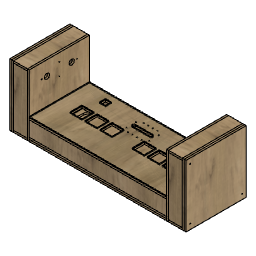
ongekicon-diy (Autodesk Fusion 360 design; units mm, degrees)
Autodesk Fusion 360 part; units mm, degrees
(part 1 of 2)
sketch "스케치1" plane through (0, 0, 0) normal (0, 0, 1) x (1, 0, 0)
  line L0 (289, -642.7336) -> (375, -642.7336)
  line L1 (375, -656.7336) -> (289, -656.7336)
  arc A0 (289, -642.7336) -> (289, -656.7336) centre (289, -649.7336) ccw
  arc A1 (375, -656.7336) -> (375, -642.7336) centre (375, -649.7336) ccw
  line L2 (289, -642.7336) -> (289, -656.7336) construction
  line L3 (375, -642.7336) -> (375, -656.7336) construction
  line L4 (375, -642.7336) -> (386.9217, -626.4866) construction
  line L5 (386.9217, -626.4866) -> (386.9217, -642.6701) construction
  line L6 (386.9217, -642.6701) -> (386.9217, -656.6701) construction
  line L7 (386.9217, -656.6701) -> (386.9217, -672.8535) construction
  line L8 (375, -656.7336) -> (386.9217, -672.8535) construction
  line L9 (386.9217, -642.6701) -> (386.9217, -656.6701) construction
  line L10 (375, -642.7336) -> (375, -656.7336) construction
  line L11 (375, -642.7336) -> (386.9217, -626.4866) construction
  line L12 (375, -656.7336) -> (386.9217, -672.8535) construction
  line L13 (386.9217, -656.6701) -> (386.9217, -672.8535) construction
  line L14 (386.9217, -626.4866) -> (386.9217, -642.6701) construction
  arc A2 (375, -656.7336) -> (375, -642.7336) centre (375, -649.7336) ccw
  line L15 (375, -642.7336) -> (386.9217, -642.7336) construction
  line L16 (289, -642.7336) -> (277.0783, -642.7336) construction
  line L17 (277.0783, -642.7336) -> (277.0783, -626.5501) construction
  line L18 (277.0783, -626.5501) -> (289, -642.7336) construction
  line L19 (289, -656.7336) -> (277.0783, -656.7336) construction
  line L20 (277.0783, -656.7336) -> (277.0783, -672.9171) construction
  line L21 (289, -656.7336) -> (277.0783, -672.9171) construction
  circle A3 centre (277.0783, -626.5501) radius 2.65
  circle A4 centre (277.0783, -672.9171) radius 2.65
  circle A5 centre (386.9217, -626.4866) radius 2.65
  circle A6 centre (386.9217, -672.8535) radius 2.65
  line L22 (299.0783, -611.6097) -> (277.0783, -626.5501) construction
  circle A7 centre (299.0783, -611.6097) radius 2.65
  line L23 (299.0783, -611.6097) -> (321.0783, -611.6097) construction
  line L24 (321.0783, -611.6097) -> (343.0783, -611.6097) construction
  line L25 (343.0783, -611.6097) -> (365.0783, -611.6097) construction
  line L26 (364.9217, -687.7939) -> (386.9217, -672.8535) construction
  line L27 (364.9217, -687.7939) -> (342.9217, -687.7939) construction
  line L28 (342.9217, -687.7939) -> (320.9217, -687.7939) construction
  line L29 (320.9217, -687.7939) -> (298.9217, -687.7939) construction
  circle A8 centre (321.0783, -611.6097) radius 2.65
  circle A9 centre (343.0783, -611.6097) radius 2.65
  circle A10 centre (365.0783, -611.6097) radius 2.65
  circle A11 centre (364.9217, -687.7939) radius 2.65
  circle A12 centre (342.9217, -687.7939) radius 2.65
  circle A13 centre (320.9217, -687.7939) radius 2.65
  circle A14 centre (298.9217, -687.7939) radius 2.65
  line L30 (0, -575) -> (664, -575)
  line L31 (664, -575) -> (664, -866)
  line L32 (664, -866) -> (0, -866)
  line L33 (0, -866) -> (0, -575)
  line L34 (0, -575) -> (332, -575) construction
  line L35 (332, -575) -> (332, -649.7336) construction
  line L36 (0, -649.7336) -> (0, -575) construction
  line L37 (332, -649.7336) -> (289, -649.7336) construction
  line L38 (150.8081, -749.0793) -> (137.915, -749.0793) construction
  line L39 (223.7013, -749.0793) -> (210.8081, -749.0793) construction
  line L40 (0, -1260) -> (664, -1260)
  line L41 (664, -1260) -> (664, -1333)
  line L42 (664, -1333) -> (0, -1333)
  line L43 (0, -1333) -> (0, -1260)
  line L44 (0, -1495) -> (0, -1422)
  line L45 (664, -1422) -> (664, -1495)
  line L46 (0, -1422) -> (664, -1422)
  line L47 (664, -1495) -> (0, -1495)
  line L48 (664, 150) -> (664, -141)
  line L49 (0, -141) -> (0, 150)
  line L50 (664, -141) -> (0, -141)
  line L51 (604, 120) -> (60, 120)
  line L52 (634, -81) -> (634, 90)
  line L53 (30, 90) -> (30, -81)
  line L54 (634, 120) -> (30, -111) construction
  line L55 (60, -111) -> (604, -111)
  line L56 (0, 150) -> (664, 150)
  line L57 (30, 120) -> (634, -111) construction
  line L58 (0, 120) -> (0, 150) construction
  line L59 (664, -141) -> (644.0002, -121.0002) construction
  line L60 (664, 150) -> (644.0002, 130.0002) construction
  line L61 (0, 150) -> (19.9998, 130.0002) construction
  line L62 (0, -141) -> (19.9998, -121.0002) construction
  line L63 (664, -491) -> (644.0002, -471.0002) construction
  line L64 (664, -200) -> (644.0002, -219.9998) construction
  line L65 (634, -431) -> (634, -260)
  line L66 (664, -200) -> (664, -491)
  line L67 (30, -230) -> (634, -461) construction
  line L68 (0, -200) -> (664, -200)
  line L69 (60, -461) -> (604, -461)
  line L70 (664, -491) -> (0, -491)
  line L71 (634, -230) -> (30, -461) construction
  line L72 (30, -260) -> (30, -431)
  line L73 (0, -491) -> (19.9998, -471.0002) construction
  line L74 (604, -230) -> (60, -230)
  line L75 (0, -491) -> (0, -200)
  line L76 (0, -200) -> (19.9998, -219.9998) construction
  line L77 (0, -230) -> (0, -200) construction
  arc A15 (60, 120) -> (30, 90) centre (60, 90) ccw
  arc A16 (634, 90) -> (604, 120) centre (604, 90) ccw
  arc A17 (604, -111) -> (634, -81) centre (604, -81) ccw
  arc A18 (30, -81) -> (60, -111) centre (60, -81) ccw
  arc A19 (60, -230) -> (30, -260) centre (60, -260) ccw
  arc A20 (634, -260) -> (604, -230) centre (604, -260) ccw
  arc A21 (604, -461) -> (634, -431) centre (604, -431) ccw
  arc A22 (30, -431) -> (60, -461) centre (60, -431) ccw
  circle A23 centre (644.0002, -219.9998) radius 3.25
  circle A24 centre (644.0002, -471.0002) radius 3.25
  circle A25 centre (644.0002, -121.0002) radius 9
  circle A26 centre (644.0002, 130.0002) radius 9
  circle A27 centre (19.9998, 130.0002) radius 9
  circle A28 centre (19.9998, -121.0002) radius 9
  circle A29 centre (19.9998, -219.9998) radius 3.25
  circle A30 centre (19.9998, -471.0002) radius 3.25
  line L78 (664, -575) -> (644, -575) construction
  line L79 (644, -575) -> (644, -595) construction
  line L80 (644, -595) -> (664, -595) construction
  line L81 (664, -595) -> (664, -575) construction
  line L82 (664, -866) -> (644, -866) construction
  line L83 (644, -866) -> (644, -846) construction
  line L84 (644, -846) -> (664, -846) construction
  line L85 (664, -846) -> (664, -866) construction
  line L86 (0, -866) -> (20, -866) construction
  line L87 (20, -866) -> (20, -846) construction
  line L88 (20, -846) -> (0, -846) construction
  line L89 (0, -846) -> (0, -866) construction
  line L90 (0, -575) -> (20, -575) construction
  line L91 (20, -575) -> (20, -595) construction
  line L92 (20, -595) -> (0, -595) construction
  line L93 (0, -595) -> (0, -575) construction
  circle A31 centre (20, -595) radius 2.5 construction
  circle A32 centre (644, -595) radius 2.5 construction
  circle A33 centre (20, -846) radius 2.5 construction
  circle A34 centre (644, -846) radius 2.5 construction
  line L94 (1066.4968, -1645.2647) -> (1357.4968, -1645.2647)
  line L95 (1357.4968, -1645.2647) -> (1357.4968, -1712.2647)
  line L96 (1357.4968, -1712.2647) -> (1066.4968, -1712.2647)
  line L97 (1066.4968, -1712.2647) -> (1066.4968, -1645.2647)
  line L98 (716.4968, -1645.2647) -> (1007.4968, -1645.2647)
  line L99 (1007.4968, -1645.2647) -> (1007.4968, -1712.2647)
  line L100 (1007.4968, -1712.2647) -> (716.4968, -1712.2647)
  line L101 (716.4968, -1712.2647) -> (716.4968, -1645.2647)
  line L102 (1066.4968, -845.2647) -> (1357.4968, -845.2647)
  line L103 (1357.4968, -845.2647) -> (1357.4968, -912.2647)
  line L104 (1357.4968, -912.2647) -> (1066.4968, -912.2647)
  line L105 (1066.4968, -912.2647) -> (1066.4968, -845.2647)
  line L106 (716.4968, -845.2647) -> (1007.4968, -845.2647)
  line L107 (1007.4968, -845.2647) -> (1007.4968, -912.2647)
  line L108 (1007.4968, -912.2647) -> (716.4968, -912.2647)
  line L109 (716.4968, -912.2647) -> (716.4968, -845.2647)
  line L110 (1406.0943, -1345.433) -> (1473.0943, -1345.433)
  line L111 (1473.0943, -1345.433) -> (1473.0943, -1627.433)
  line L112 (1473.0943, -1627.433) -> (1406.0943, -1627.433)
  line L113 (1406.0943, -1627.433) -> (1406.0943, -1345.433)
  line L114 (1573.0943, -1627.433) -> (1506.0943, -1627.433)
  line L115 (1506.0943, -1627.433) -> (1506.0943, -1345.433)
  line L116 (1506.0943, -1345.433) -> (1573.0943, -1345.433)
  line L117 (1573.0943, -1345.433) -> (1573.0943, -1627.433)
  line L118 (1506.0943, -1277.433) -> (1506.0943, -995.433)
  line L119 (1506.0943, -995.433) -> (1573.0943, -995.433)
  line L120 (1573.0943, -995.433) -> (1573.0943, -1277.433)
  line L121 (1573.0943, -1277.433) -> (1506.0943, -1277.433)
  line L122 (1406.0943, -1277.433) -> (1406.0943, -995.433)
  line L123 (1406.0943, -995.433) -> (1473.0943, -995.433)
  line L124 (1473.0943, -1277.433) -> (1406.0943, -1277.433)
  line L125 (1473.0943, -995.433) -> (1473.0943, -1277.433)
  line L126 (725.4968, -1278.433) -> (716.4968, -1278.433)
  line L127 (998.4968, -1278.433) -> (725.4968, -1278.433)
  line L128 (998.4968, -1278.433) -> (1007.4968, -1278.433)
  line L129 (1007.4968, -978.433) -> (1007.4968, -1278.433)
  line L130 (1007.4968, -978.433) -> (716.4968, -978.433)
  line L131 (716.4968, -978.433) -> (716.4968, -1278.433)
  arc A35 (1661.5009, -1535.9592) -> (1691.5009, -1565.9592) centre (1691.5009, -1535.9592) ccw
  line L132 (1871.5009, -1325.9592) -> (1691.5009, -1325.9592)
  arc A36 (1691.5009, -1325.9592) -> (1661.5009, -1355.9592) centre (1691.5009, -1355.9592) ccw
  line L133 (1661.5009, -1355.9592) -> (1661.5009, -1535.9592)
  circle A37 centre (1656.0009, -1571.4592) radius 3.25
  circle A38 centre (1656.0009, -1320.4592) radius 3.25
  line L134 (1636.0009, -1295.9592) -> (1636.0009, -1595.9592)
  arc A39 (2251.5009, -1355.9592) -> (2221.5009, -1325.9592) centre (2221.5009, -1355.9592) ccw
  arc A40 (2221.5009, -1565.9592) -> (2251.5009, -1535.9592) centre (2221.5009, -1535.9592) ccw
  circle A41 centre (2257.0009, -1571.4592) radius 10
  circle A42 centre (2257.0009, -1320.4592) radius 10
  circle A43 centre (2006.0009, -1571.4592) radius 10
  line L135 (2221.5009, -1325.9592) -> (2041.5009, -1325.9592)
  circle A44 centre (2006.0009, -1320.4592) radius 10
  line L136 (2041.5009, -1565.9592) -> (2221.5009, -1565.9592)
  line L137 (2277.0009, -1295.9592) -> (2277.0009, -1595.9592)
  arc A45 (2011.5009, -1535.9592) -> (2041.5009, -1565.9592) centre (2041.5009, -1535.9592) ccw
  arc A46 (2041.5009, -1325.9592) -> (2011.5009, -1355.9592) centre (2041.5009, -1355.9592) ccw
  line L138 (2251.5009, -1535.9592) -> (2251.5009, -1355.9592)
  line L139 (2011.5009, -1355.9592) -> (2011.5009, -1535.9592)
  line L140 (1986.0009, -1295.9592) -> (1986.0009, -1595.9592)
  line L141 (1927.0009, -1295.9592) -> (1927.0009, -1595.9592)
  line L142 (1901.5009, -1535.9592) -> (1901.5009, -1355.9592)
  line L143 (1691.5009, -1565.9592) -> (1871.5009, -1565.9592)
  arc A47 (1871.5009, -1565.9592) -> (1901.5009, -1535.9592) centre (1871.5009, -1535.9592) ccw
  arc A48 (1901.5009, -1355.9592) -> (1871.5009, -1325.9592) centre (1871.5009, -1355.9592) ccw
  circle A49 centre (1907.0009, -1320.4592) radius 3.25
  circle A50 centre (1907.0009, -1571.4592) radius 3.25
  line L144 (1927.0009, -1295.9592) -> (1636.0009, -1295.9592)
  line L145 (1927.0009, -1595.9592) -> (1636.0009, -1595.9592)
  line L146 (2277.0009, -1595.9592) -> (1986.0009, -1595.9592)
  line L147 (2277.0009, -1295.9592) -> (1986.0009, -1295.9592)
  line L148 (1927.0009, -1245.9592) -> (1636.0009, -1245.9592)
  line L149 (1927.0009, -945.9592) -> (1927.0009, -1245.9592)
  line L150 (1661.5009, -1005.9592) -> (1661.5009, -1185.9592)
  line L151 (1636.0009, -945.9592) -> (1636.0009, -1245.9592)
  arc A51 (1901.5009, -1005.9592) -> (1871.5009, -975.9592) centre (1871.5009, -1005.9592) ccw
  circle A52 centre (1907.0009, -1221.4592) radius 3.25
  circle A53 centre (1656.0009, -970.4592) radius 3.25
  circle A54 centre (1907.0009, -970.4592) radius 3.25
  line L152 (2277.0009, -945.9592) -> (2277.0009, -1245.9592)
  line L153 (2041.5009, -1215.9592) -> (2221.5009, -1215.9592)
  line L154 (2277.0009, -945.9592) -> (1986.0009, -945.9592)
  line L155 (1691.5009, -1215.9592) -> (1871.5009, -1215.9592)
  line L156 (1901.5009, -1185.9592) -> (1901.5009, -1005.9592)
  arc A55 (1871.5009, -1215.9592) -> (1901.5009, -1185.9592) centre (1871.5009, -1185.9592) ccw
  line L157 (1871.5009, -975.9592) -> (1691.5009, -975.9592)
  line L158 (1986.0009, -945.9592) -> (1986.0009, -1245.9592)
  circle A56 centre (1656.0009, -1221.4592) radius 3.25
  arc A57 (1661.5009, -1185.9592) -> (1691.5009, -1215.9592) centre (1691.5009, -1185.9592) ccw
  arc A58 (1691.5009, -975.9592) -> (1661.5009, -1005.9592) centre (1691.5009, -1005.9592) ccw
  line L159 (1927.0009, -945.9592) -> (1636.0009, -945.9592)
  arc A59 (2011.5009, -1185.9592) -> (2041.5009, -1215.9592) centre (2041.5009, -1185.9592) ccw
  circle A60 centre (2257.0009, -970.4592) radius 10
  circle A61 centre (2006.0009, -1221.4592) radius 10
  line L160 (2011.5009, -1005.9592) -> (2011.5009, -1185.9592)
  arc A62 (2041.5009, -975.9592) -> (2011.5009, -1005.9592) centre (2041.5009, -1005.9592) ccw
  circle A63 centre (2257.0009, -1221.4592) radius 10
  circle A64 centre (2006.0009, -970.4592) radius 10
  line L161 (2277.0009, -1245.9592) -> (1986.0009, -1245.9592)
  line L162 (2251.5009, -1185.9592) -> (2251.5009, -1005.9592)
  arc A65 (2221.5009, -1215.9592) -> (2251.5009, -1185.9592) centre (2221.5009, -1185.9592) ccw
  line L163 (2221.5009, -975.9592) -> (2041.5009, -975.9592)
  arc A66 (2251.5009, -1005.9592) -> (2221.5009, -975.9592) centre (2221.5009, -1005.9592) ccw
  line L164 (716.4968, -1317.433) -> (716.4968, -1617.433)
  circle A67 centre (801.9968, -1386.933) radius 12.5
  line L165 (1007.4968, -1317.433) -> (716.4968, -1317.433)
  line L166 (1007.4968, -1617.433) -> (716.4968, -1617.433)
  circle A68 centre (921.9968, -1386.933) radius 12.5
  line L167 (716.4968, -1521.933) -> (716.4968, -1617.433)
  circle A69 centre (946.9968, -1386.933) radius 2.2361
  circle A70 centre (776.9968, -1386.933) radius 2.2592
  circle A71 centre (861.9968, -1416.933) radius 2.2361
  line L168 (1007.4968, -1317.433) -> (1007.4968, -1617.433)
  line L169 (1007.4968, -1521.933) -> (716.4968, -1521.933) construction
  circle A72 centre (861.9968, -1356.933) radius 2.2361
  line L170 (716.4968, -1278.433) -> (736.4968, -1278.433) construction
  line L171 (736.4968, -1278.433) -> (736.4968, -1253.933) construction
  line L172 (736.4968, -1253.933) -> (716.4968, -1253.933) construction
  line L173 (716.4968, -1253.933) -> (716.4968, -1278.433) construction
  line L174 (1007.4968, -1278.433) -> (987.4968, -1278.433) construction
  line L175 (987.4968, -1278.433) -> (987.4968, -1253.933) construction
  line L176 (987.4968, -1253.933) -> (1007.4968, -1253.933) construction
  line L177 (1007.4968, -1253.933) -> (1007.4968, -1278.433) construction
  line L178 (1007.4968, -978.433) -> (987.4968, -978.433) construction
  line L179 (987.4968, -978.433) -> (987.4968, -1002.933) construction
  line L180 (987.4968, -1002.933) -> (1007.4968, -1002.933) construction
  line L181 (1007.4968, -1002.933) -> (1007.4968, -978.433) construction
  circle A73 centre (736.4968, -1253.933) radius 2.5
  circle A74 centre (987.4968, -1253.933) radius 2.5
  circle A75 centre (987.4968, -1002.933) radius 2.5
  circle A76 centre (1086.4968, -1002.933) radius 2.5
  line L182 (1086.4968, -1278.433) -> (1086.4968, -1253.933) construction
  line L183 (1066.4968, -978.433) -> (1066.4968, -1278.433)
  line L184 (1066.4968, -1002.933) -> (1066.4968, -978.433) construction
  line L185 (1337.4968, -1002.933) -> (1357.4968, -1002.933) construction
  line L186 (1337.4968, -1253.933) -> (1357.4968, -1253.933) construction
  line L187 (1066.4968, -1253.933) -> (1066.4968, -1278.433) construction
  line L188 (1086.4968, -1253.933) -> (1066.4968, -1253.933) construction
  circle A77 centre (1086.4968, -1253.933) radius 2.5
  line L189 (1066.4968, -1278.433) -> (1086.4968, -1278.433) construction
  line L190 (1348.4968, -1278.433) -> (1357.4968, -1278.433)
  line L191 (1086.4968, -1002.933) -> (1066.4968, -1002.933) construction
  line L192 (1066.4968, -978.433) -> (1086.4968, -978.433) construction
  line L193 (1357.4968, -1253.933) -> (1357.4968, -1278.433) construction
  line L194 (1357.4968, -1002.933) -> (1357.4968, -978.433) construction
  line L195 (1337.4968, -978.433) -> (1337.4968, -1002.933) construction
  line L196 (1348.4968, -1278.433) -> (1075.4968, -1278.433)
  line L197 (1086.4968, -978.433) -> (1086.4968, -1002.933) construction
  line L198 (1357.4968, -978.433) -> (1337.4968, -978.433) construction
  line L199 (1357.4968, -978.433) -> (1066.4968, -978.433)
  line L200 (1357.4968, -978.433) -> (1357.4968, -1278.433)
  line L201 (1357.4968, -1278.433) -> (1337.4968, -1278.433) construction
  line L202 (1075.4968, -1278.433) -> (1066.4968, -1278.433)
  circle A78 centre (1337.4968, -1253.933) radius 2.5
  circle A79 centre (1337.4968, -1002.933) radius 2.5
  line L203 (1337.4968, -1278.433) -> (1337.4968, -1253.933) construction
  line L204 (0, -1260) -> (166, -1260) construction
  line L205 (166, -1260) -> (166, -1297.5) construction
  line L206 (166, -1297.5) -> (0, -1297.5) construction
  line L207 (0, -1297.5) -> (0, -1260) construction
  line L208 (664, -1260) -> (498, -1260) construction
  line L209 (498, -1260) -> (498, -1297.5) construction
  line L210 (498, -1297.5) -> (664, -1297.5) construction
  line L211 (664, -1297.5) -> (664, -1260) construction
  circle A80 centre (456.3298, -1576.2079) radius 4
  circle A81 centre (547.3298, -1605.2079) radius 4
  line L212 (592.8298, -1576.2079) -> (592.8298, -1605.2079) construction
  circle A82 centre (592.8298, -1590.7079) radius 4
  circle A83 centre (547.3298, -1576.2079) radius 4
  line L213 (410.8298, -1576.2079) -> (592.8298, -1576.2079) construction
  line L214 (365.3298, -1605.2079) -> (365.3298, -1627.2079) construction
  line L215 (410.8298, -1605.2079) -> (365.3298, -1605.2079) construction
  line L216 (410.8298, -1627.2079) -> (410.8298, -1605.2079) construction
  line L217 (410.8298, -1605.2079) -> (410.8298, -1576.2079) construction
  circle A84 centre (410.8298, -1590.7079) radius 4
  circle A85 centre (501.8298, -1590.7079) radius 4
  line L218 (365.3298, -1627.2079) -> (410.8298, -1627.2079) construction
  circle A86 centre (456.3298, -1605.2079) radius 4
  line L219 (592.8298, -1605.2079) -> (410.8298, -1605.2079) construction
  line L220 (592.8298, -1576.2079) -> (638.3298, -1576.2079) construction
  line L221 (638.3298, -1576.2079) -> (638.3298, -1554.2079) construction
  line L222 (638.3298, -1554.2079) -> (592.8298, -1554.2079) construction
  line L223 (592.8298, -1554.2079) -> (592.8298, -1576.2079) construction
  line L224 (521.8298, -1571.2079) -> (481.2298, -1571.2079)
  line L225 (479.3298, -1573.1079) -> (479.3298, -1578.7079)
  line L226 (481.8298, -1581.2079) -> (521.8298, -1581.2079)
  line L227 (524.3298, -1578.7079) -> (524.3298, -1573.7079)
  arc A87 (524.3298, -1573.7079) -> (521.8298, -1571.2079) centre (521.8298, -1573.7079) ccw
  arc A88 (521.8298, -1581.2079) -> (524.3298, -1578.7079) centre (521.8298, -1578.7079) ccw
  arc A89 (479.3298, -1578.7079) -> (481.8298, -1581.2079) centre (481.8298, -1578.7079) ccw
  arc A90 (481.2298, -1571.2079) -> (479.3298, -1573.1079) centre (481.2298, -1573.1079) ccw
  line L228 (365.3298, -1554.2079) -> (638.3298, -1554.2079)
  line L229 (638.3298, -1554.2079) -> (638.3298, -1627.2079)
  line L230 (638.3298, -1627.2079) -> (365.3298, -1627.2079)
  line L231 (365.3298, -1627.2079) -> (365.3298, -1554.2079)
  arc A91 (884.4968, -1545.933) -> (881.9968, -1543.433) centre (881.9968, -1545.933) ccw
  line L232 (884.4968, -1550.933) -> (884.4968, -1545.933)
  line L233 (770.9968, -1577.433) -> (770.9968, -1548.433) construction
  line L234 (881.9968, -1543.433) -> (841.3968, -1543.433)
  arc A92 (881.9968, -1553.433) -> (884.4968, -1550.933) centre (881.9968, -1550.933) ccw
  arc A93 (839.4968, -1550.933) -> (841.9968, -1553.433) centre (841.9968, -1550.933) ccw
  circle A94 centre (816.4968, -1577.433) radius 4
  circle A95 centre (861.9968, -1562.933) radius 4
  line L235 (841.9968, -1553.433) -> (881.9968, -1553.433)
  arc A96 (841.3968, -1543.433) -> (839.4968, -1545.333) centre (841.3968, -1545.333) ccw
  circle A97 centre (816.4968, -1548.433) radius 4
  line L236 (952.9968, -1577.433) -> (770.9968, -1577.433) construction
  line L237 (839.4968, -1545.333) -> (839.4968, -1550.933)
  line L238 (770.9968, -1548.433) -> (952.9968, -1548.433) construction
  circle A98 centre (770.9968, -1562.933) radius 4
  circle A99 centre (952.9968, -1562.933) radius 4
  circle A100 centre (907.4968, -1577.433) radius 4
  circle A101 centre (907.4968, -1548.433) radius 4
  line L239 (952.9968, -1548.433) -> (952.9968, -1577.433) construction
  line L240 (952.9968, -1548.433) -> (1007.4968, -1548.433) construction
  line L241 (1007.4968, -1548.433) -> (1007.4968, -1521.933) construction
  line L242 (1007.4968, -1521.933) -> (952.9968, -1521.933) construction
  line L243 (952.9968, -1521.933) -> (952.9968, -1548.433) construction
  line L244 (770.9968, -1577.433) -> (716.4968, -1577.433) construction
  line L245 (716.4968, -1577.433) -> (716.4968, -1594.933) construction
  line L246 (716.4968, -1594.933) -> (770.9968, -1594.933) construction
  line L247 (770.9968, -1594.933) -> (770.9968, -1577.433) construction
  circle A102 centre (1302.9968, -1562.933) radius 4
  circle A103 centre (1257.4968, -1548.433) radius 4
  line L248 (1357.4968, -1521.933) -> (1302.9968, -1521.933) construction
  arc A104 (1231.9968, -1553.433) -> (1234.4968, -1550.933) centre (1231.9968, -1550.933) ccw
  arc A105 (1234.4968, -1545.933) -> (1231.9968, -1543.433) centre (1231.9968, -1545.933) ccw
  line L249 (1120.9968, -1577.433) -> (1120.9968, -1548.433) construction
  line L250 (1231.9968, -1543.433) -> (1191.3968, -1543.433)
  line L251 (1120.9968, -1603.933) -> (1120.9968, -1577.433) construction
  circle A106 centre (1211.9968, -1562.933) radius 4
  line L252 (1302.9968, -1521.933) -> (1302.9968, -1548.433) construction
  line L253 (1302.9968, -1548.433) -> (1302.9968, -1577.433) construction
  circle A107 centre (1257.4968, -1577.433) radius 4
  line L254 (1357.4968, -1317.433) -> (1357.4968, -1617.433)
  line L255 (1302.9968, -1548.433) -> (1357.4968, -1548.433) construction
  line L256 (1357.4968, -1548.433) -> (1357.4968, -1521.933) construction
  arc A108 (1189.4968, -1550.933) -> (1191.9968, -1553.433) centre (1191.9968, -1550.933) ccw
  circle A109 centre (1120.9968, -1562.933) radius 4
  line L257 (1234.4968, -1550.933) -> (1234.4968, -1545.933)
  circle A110 centre (1211.9968, -1356.933) radius 2.2361
  circle A111 centre (1166.4968, -1548.433) radius 4
  arc A112 (1191.3968, -1543.433) -> (1189.4968, -1545.333) centre (1191.3968, -1545.333) ccw
  line L258 (1189.4968, -1545.333) -> (1189.4968, -1550.933)
  circle A113 centre (1166.4968, -1577.433) radius 4
  circle A114 centre (1211.9968, -1416.933) radius 2.2361
  circle A115 centre (1126.9968, -1386.933) radius 2.2592
  line L259 (1191.9968, -1553.433) -> (1231.9968, -1553.433)
  circle A116 centre (1151.9968, -1386.933) radius 12.5
  line L260 (1357.4968, -1617.433) -> (1066.4968, -1617.433)
  line L261 (1120.9968, -1577.433) -> (1066.4968, -1577.433) construction
  line L262 (1066.4968, -1603.933) -> (1120.9968, -1603.933) construction
  line L263 (1066.4968, -1521.933) -> (1066.4968, -1617.433)
  line L264 (1066.4968, -1577.433) -> (1066.4968, -1603.933) construction
  line L265 (1066.4968, -1317.433) -> (1066.4968, -1617.433)
  line L266 (1302.9968, -1577.433) -> (1120.9968, -1577.433) construction
  line L267 (1357.4968, -1317.433) -> (1066.4968, -1317.433)
  line L268 (1120.9968, -1548.433) -> (1302.9968, -1548.433) construction
  line L269 (1357.4968, -1521.933) -> (1066.4968, -1521.933) construction
  circle A117 centre (1296.9968, -1386.933) radius 2.2361
  circle A118 centre (1271.9968, -1386.933) radius 12.5
  line L270 (278.3298, -1554.2079) -> (232.8298, -1554.2079) construction
  line L271 (121.8298, -1581.2079) -> (161.8298, -1581.2079)
  line L272 (161.8298, -1571.2079) -> (121.2298, -1571.2079)
  line L273 (50.8298, -1576.2079) -> (232.8298, -1576.2079) construction
  line L274 (119.3298, -1573.1079) -> (119.3298, -1578.7079)
  line L275 (278.3298, -1554.2079) -> (278.3298, -1627.2079)
  line L276 (232.8298, -1576.2079) -> (232.8298, -1605.2079) construction
  line L277 (278.3298, -1576.2079) -> (278.3298, -1554.2079) construction
  arc A119 (161.8298, -1581.2079) -> (164.3298, -1578.7079) centre (161.8298, -1578.7079) ccw
  arc A120 (119.3298, -1578.7079) -> (121.8298, -1581.2079) centre (121.8298, -1578.7079) ccw
  line L278 (232.8298, -1554.2079) -> (232.8298, -1576.2079) construction
  line L279 (232.8298, -1576.2079) -> (278.3298, -1576.2079) construction
  circle A121 centre (187.3298, -1576.2079) radius 4
  arc A122 (121.2298, -1571.2079) -> (119.3298, -1573.1079) centre (121.2298, -1573.1079) ccw
  line L280 (164.3298, -1578.7079) -> (164.3298, -1573.7079)
  circle A123 centre (187.3298, -1605.2079) radius 4
  circle A124 centre (141.8298, -1590.7079) radius 4
  arc A125 (164.3298, -1573.7079) -> (161.8298, -1571.2079) centre (161.8298, -1573.7079) ccw
  line L281 (278.3298, -1627.2079) -> (5.3298, -1627.2079)
  circle A126 centre (96.3298, -1576.2079) radius 4
  line L282 (232.8298, -1605.2079) -> (50.8298, -1605.2079) construction
  circle A127 centre (232.8298, -1590.7079) radius 4
  line L283 (50.8298, -1605.2079) -> (5.3298, -1605.2079) construction
  line L284 (5.3298, -1627.2079) -> (5.3298, -1554.2079)
  circle A128 centre (50.8298, -1590.7079) radius 4
  line L285 (50.8298, -1627.2079) -> (50.8298, -1605.2079) construction
  line L286 (5.3298, -1627.2079) -> (50.8298, -1627.2079) construction
  line L287 (50.8298, -1605.2079) -> (50.8298, -1576.2079) construction
  circle A129 centre (96.3298, -1605.2079) radius 4
  line L288 (5.3298, -1554.2079) -> (278.3298, -1554.2079)
  line L289 (5.3298, -1605.2079) -> (5.3298, -1627.2079) construction
  line L290 (138.1898, -635.6975) -> (109.1898, -635.6975)
  line L291 (109.1898, -635.6975) -> (109.1898, -606.6975)
  line L292 (109.1898, -606.6975) -> (138.1898, -606.6975)
  line L293 (138.1898, -606.6975) -> (138.1898, -635.6975)
  line L294 (138.1898, -635.6975) -> (109.1898, -606.6975) construction
  line L295 (109.1898, -635.6975) -> (138.1898, -606.6975) construction
  line L296 (525.8102, -635.6975) -> (554.8102, -635.6975)
  line L297 (554.8102, -635.6975) -> (554.8102, -606.6975)
  line L298 (554.8102, -606.6975) -> (525.8102, -606.6975)
  line L299 (525.8102, -606.6975) -> (525.8102, -635.6975)
  line L300 (525.8102, -635.6975) -> (554.8102, -606.6975) construction
  line L301 (554.8102, -635.6975) -> (525.8102, -606.6975) construction
  line L302 (664, -1216) -> (644, -1216) construction
  line L303 (644, -945) -> (664, -945) construction
  circle A130 centre (644, -1196) radius 2.5 construction
  line L304 (644, -1216) -> (644, -1196) construction
  line L305 (554.8102, -985.6975) -> (525.8102, -956.6975) construction
  line L306 (554.8102, -985.6975) -> (554.8102, -956.6975)
  line L307 (664, -925) -> (644, -925) construction
  line L308 (109.1898, -985.6975) -> (109.1898, -956.6975)
  line L309 (0, -925) -> (20, -925) construction
  line L310 (20, -925) -> (20, -945) construction
  line L311 (138.1898, -956.6975) -> (138.1898, -985.6975)
  line L312 (0, -999.7336) -> (0, -925) construction
  line L313 (525.8102, -956.6975) -> (525.8102, -985.6975)
  line L314 (525.8102, -985.6975) -> (554.8102, -956.6975) construction
  line L315 (525.8102, -985.6975) -> (554.8102, -985.6975)
  circle A131 centre (644, -945) radius 2.5 construction
  line L316 (664, -945) -> (664, -925) construction
  line L317 (664, -925) -> (664, -1216)
  line L318 (644, -925) -> (644, -945) construction
  circle A132 centre (20, -1196) radius 2.5 construction
  line L319 (0, -1216) -> (0, -925)
  line L320 (0, -945) -> (0, -925) construction
  line L321 (109.1898, -956.6975) -> (138.1898, -956.6975)
  line L322 (0, -925) -> (332, -925) construction
  line L323 (0, -1216) -> (20, -1216) construction
  line L324 (20, -1196) -> (0, -1196) construction
  line L325 (0, -1196) -> (0, -1216) construction
  line L326 (20, -1216) -> (20, -1196) construction
  arc A133 (289, -992.7336) -> (289, -1006.7336) centre (289, -999.7336) ccw
  arc A134 (375, -1006.7336) -> (375, -992.7336) centre (375, -999.7336) ccw
  arc A135 (375, -1006.7336) -> (375, -992.7336) centre (375, -999.7336) ccw
  line L327 (138.1898, -985.6975) -> (109.1898, -985.6975)
  circle A136 centre (20, -945) radius 2.5 construction
  line L328 (20, -945) -> (0, -945) construction
  line L329 (109.1898, -985.6975) -> (138.1898, -956.6975) construction
  line L330 (138.1898, -985.6975) -> (109.1898, -956.6975) construction
  line L331 (375, -1006.7336) -> (289, -1006.7336)
  line L332 (664, -1216) -> (0, -1216)
  line L333 (0, -925) -> (664, -925)
  line L334 (289, -992.7336) -> (375, -992.7336)
  line L335 (644, -1196) -> (664, -1196) construction
  line L336 (664, -1196) -> (664, -1216) construction
  line L337 (554.8102, -956.6975) -> (525.8102, -956.6975)
  line L338 (644, 525) -> (644, 505) construction
  circle A137 centre (644, 254) radius 2.5
  line L339 (664, 525) -> (644, 525) construction
  line L340 (644, 505) -> (664, 505) construction
  line L341 (664, 254) -> (664, 234) construction
  line L342 (664, 505) -> (664, 525) construction
  circle A138 centre (644, 505) radius 2.5
  line L343 (644, 234) -> (644, 254) construction
  line L344 (664, 234) -> (644, 234) construction
  line L345 (644, 254) -> (664, 254) construction
  line L346 (664, 525) -> (664, 234)
  line L347 (0, 525) -> (332, 525) construction
  line L348 (0, 525) -> (664, 525)
  line L349 (664, 234) -> (0, 234)
  line L350 (0, 234) -> (0, 525)
  line L351 (20, 234) -> (20, 254) construction
  line L352 (20, 254) -> (0, 254) construction
  line L353 (0, 254) -> (0, 234) construction
  line L354 (0, 234) -> (20, 234) construction
  circle A139 centre (20, 254) radius 2.5
  circle A140 centre (20, 505) radius 2.5
  line L355 (0, 525) -> (20, 525) construction
  line L356 (20, 505) -> (0, 505) construction
  line L357 (20, 525) -> (20, 505) construction
  line L358 (0, 505) -> (0, 525) construction
  line L359 (180.5, -1312) -> (151.5, -1312)
  line L360 (151.5, -1312) -> (151.5, -1283)
  line L361 (151.5, -1283) -> (180.5, -1283)
  line L362 (180.5, -1283) -> (180.5, -1312)
  line L363 (180.5, -1312) -> (151.5, -1283) construction
  line L364 (151.5, -1312) -> (180.5, -1283) construction
  line L365 (318.75, -1303.75) -> (306.25, -1303.75)
  line L366 (306.25, -1303.75) -> (306.25, -1291.25)
  line L367 (306.25, -1291.25) -> (318.75, -1291.25)
  line L368 (318.75, -1291.25) -> (318.75, -1303.75)
  line L369 (318.75, -1303.75) -> (306.25, -1291.25) construction
  line L370 (306.25, -1303.75) -> (318.75, -1291.25) construction
  line L371 (332, -1333) -> (332, -1260) construction
  line L372 (483.5, -1312) -> (512.5, -1312)
  line L373 (512.5, -1312) -> (512.5, -1283)
  line L374 (483.5, -1283) -> (483.5, -1312)
  line L375 (512.5, -1283) -> (483.5, -1283)
  line L376 (357.75, -1303.75) -> (357.75, -1291.25)
  line L377 (357.75, -1291.25) -> (345.25, -1291.25)
  line L378 (345.25, -1303.75) -> (357.75, -1303.75)
  line L379 (345.25, -1291.25) -> (345.25, -1303.75)
  line L380 (136.915, -748.0793) -> (78.915, -748.0793)
  line L381 (78.915, -748.0793) -> (78.915, -690.0793)
  line L382 (78.915, -690.0793) -> (136.915, -690.0793)
  line L383 (136.915, -690.0793) -> (136.915, -748.0793)
  line L384 (136.915, -748.0793) -> (78.915, -690.0793) construction
  line L385 (78.915, -748.0793) -> (136.915, -690.0793) construction
  line L386 (209.8081, -748.0793) -> (151.8081, -748.0793)
  line L387 (151.8081, -748.0793) -> (151.8081, -690.0793)
  line L388 (151.8081, -690.0793) -> (209.8081, -690.0793)
  line L389 (209.8081, -690.0793) -> (209.8081, -748.0793)
  line L390 (209.8081, -748.0793) -> (151.8081, -690.0793) construction
  line L391 (151.8081, -748.0793) -> (209.8081, -690.0793) construction
  line L392 (282.7013, -748.0793) -> (224.7013, -748.0793)
  line L393 (224.7013, -748.0793) -> (224.7013, -690.0793)
  line L394 (224.7013, -690.0793) -> (282.7013, -690.0793)
  line L395 (282.7013, -690.0793) -> (282.7013, -748.0793)
  line L396 (282.7013, -748.0793) -> (224.7013, -690.0793) construction
  line L397 (224.7013, -748.0793) -> (282.7013, -690.0793) construction
  line L398 (512.1919, -690.0793) -> (454.1919, -690.0793)
  line L399 (454.1919, -748.0793) -> (512.1919, -690.0793) construction
  line L400 (527.085, -748.0793) -> (585.085, -748.0793)
  line L401 (512.1919, -748.0793) -> (454.1919, -690.0793) construction
  line L402 (513.1919, -749.0793) -> (526.085, -749.0793) construction
  line L403 (454.1919, -748.0793) -> (512.1919, -748.0793)
  line L404 (585.085, -748.0793) -> (585.085, -690.0793)
  line L405 (381.2987, -690.0793) -> (381.2987, -748.0793)
  line L406 (381.2987, -748.0793) -> (439.2987, -748.0793)
  line L407 (454.1919, -690.0793) -> (454.1919, -748.0793)
  line L408 (527.085, -748.0793) -> (585.085, -690.0793) construction
  line L409 (585.085, -690.0793) -> (527.085, -690.0793)
  line L410 (439.2987, -690.0793) -> (381.2987, -690.0793)
  line L411 (381.2987, -748.0793) -> (439.2987, -690.0793) construction
  line L412 (440.2987, -749.0793) -> (453.1919, -749.0793) construction
  line L413 (585.085, -748.0793) -> (527.085, -690.0793) construction
  line L414 (527.085, -690.0793) -> (527.085, -748.0793)
  line L415 (512.1919, -748.0793) -> (512.1919, -690.0793)
  line L416 (439.2987, -748.0793) -> (381.2987, -690.0793) construction
  line L417 (439.2987, -748.0793) -> (439.2987, -690.0793)
  line L418 (225.4513, -1098.8293) -> (283.4513, -1040.8293) construction
  line L419 (152.5581, -1098.8293) -> (152.5581, -1040.8293)
  line L420 (79.665, -1098.8293) -> (79.665, -1040.8293)
  line L421 (79.665, -1040.8293) -> (137.665, -1040.8293)
  line L422 (137.665, -1098.8293) -> (79.665, -1040.8293) construction
  line L423 (152.5581, -1040.8293) -> (210.5581, -1040.8293)
  line L424 (151.5581, -1099.8293) -> (138.665, -1099.8293) construction
  line L425 (137.665, -1040.8293) -> (137.665, -1098.8293)
  line L426 (79.665, -1098.8293) -> (137.665, -1040.8293) construction
  line L427 (152.5581, -1098.8293) -> (210.5581, -1040.8293) construction
  line L428 (210.5581, -1098.8293) -> (152.5581, -1098.8293)
  line L429 (210.5581, -1098.8293) -> (152.5581, -1040.8293) construction
  line L430 (137.665, -1098.8293) -> (79.665, -1098.8293)
  line L431 (210.5581, -1040.8293) -> (210.5581, -1098.8293)
  line L432 (225.4513, -1098.8293) -> (225.4513, -1040.8293)
  line L433 (283.4513, -1098.8293) -> (225.4513, -1098.8293)
  line L434 (225.4513, -1040.8293) -> (283.4513, -1040.8293)
  line L435 (283.4513, -1040.8293) -> (283.4513, -1098.8293)
  line L436 (283.4513, -1098.8293) -> (225.4513, -1040.8293) construction
  line L437 (224.4513, -1099.8293) -> (211.5581, -1099.8293) construction
  line L438 (332, -925) -> (332, -1216) construction
  line L439 (526.335, -1098.8293) -> (584.335, -1098.8293)
  line L440 (526.335, -1040.8293) -> (526.335, -1098.8293)
  line L441 (526.335, -1098.8293) -> (584.335, -1040.8293) construction
  line L442 (380.5487, -1040.8293) -> (380.5487, -1098.8293)
  line L443 (380.5487, -1098.8293) -> (438.5487, -1098.8293)
  line L444 (439.5487, -1099.8293) -> (452.4419, -1099.8293) construction
  line L445 (453.4419, -1040.8293) -> (453.4419, -1098.8293)
  line L446 (438.5487, -1098.8293) -> (380.5487, -1040.8293) construction
  line L447 (438.5487, -1098.8293) -> (438.5487, -1040.8293)
  line L448 (380.5487, -1098.8293) -> (438.5487, -1040.8293) construction
  line L449 (438.5487, -1040.8293) -> (380.5487, -1040.8293)
  line L450 (511.4419, -1098.8293) -> (511.4419, -1040.8293)
  line L451 (584.335, -1098.8293) -> (526.335, -1040.8293) construction
  line L452 (453.4419, -1098.8293) -> (511.4419, -1098.8293)
  line L453 (584.335, -1098.8293) -> (584.335, -1040.8293)
  line L454 (511.4419, -1098.8293) -> (453.4419, -1040.8293) construction
  line L455 (511.4419, -1040.8293) -> (453.4419, -1040.8293)
  line L456 (512.4419, -1099.8293) -> (525.335, -1099.8293) construction
  line L457 (584.335, -1040.8293) -> (526.335, -1040.8293)
  line L458 (453.4419, -1098.8293) -> (511.4419, -1040.8293) construction
  line L459 (1636.0009, -945.9592) -> (1656.0009, -970.4592)
  line L460 (1656.0009, -970.4592) -> (1656.0009, -945.9592)
  circle A141 centre (736.4968, -1002.933) radius 2.6
  point P0 (332, 4.5)
  point P1 (332, 4.5)
  point P2 (332, -345.5)
  point P3 (332, -345.5)
  point P4 (0, -350)
  point P5 (1781.5009, -1445.9592)
  point P6 (2131.5009, -1445.9592)
  point P7 (2131.5009, -1095.9592)
  point P8 (1781.5009, -1095.9592)
  point P9 (861.9968, -1564.433)
  point P10 (861.9968, -1564.433)
  point P11 (166, -1297.5)
  point P12 (498, -1297.5)
  point P13 (166, -1297.5)
  point P14 (498, -1297.5)
  point P15 (501.8298, -1590.7079)
  point P16 (501.8298, -1576.2079)
  point P17 (861.9968, -1548.433)
  point P18 (861.9968, -1562.933)
  point P19 (1211.9968, -1564.433)
  point P20 (1211.9968, -1548.433)
  point P21 (1211.9968, -1562.933)
  point P22 (1211.9968, -1564.433)
  point P23 (141.8298, -1576.2079)
  point P24 (141.8298, -1590.7079)
  point P25 (540.3102, -621.1975)
  point P26 (253.7013, -719.0793)
  point P27 (107.915, -719.0793)
  point P28 (123.6898, -621.1975)
  point P29 (107.915, -719.0793)
  point P30 (253.7013, -719.0793)
  point P31 (123.6898, -621.1975)
  point P32 (540.3102, -621.1975)
  point P33 (123.6898, -621.1975)
  point P34 (540.3102, -621.1975)
  point P35 (123.6898, -971.1975)
  point P36 (540.3102, -971.1975)
  point P37 (123.6898, -971.1975)
  point P38 (540.3102, -971.1975)
  point P39 (540.3102, -971.1975)
  point P40 (123.6898, -971.1975)
  point P41 (166, -1297.5)
  point P42 (312.5, -1297.5)
  point P43 (312.5, -1297.5)
  point P44 (107.915, -719.0793)
  point P45 (180.8081, -719.0793)
  point P46 (253.7013, -719.0793)
  point P47 (556.085, -719.0793)
  point P48 (410.2987, -719.0793)
  point P49 (556.085, -719.0793)
  point P50 (410.2987, -719.0793)
  point P51 (410.2987, -719.0793)
  point P52 (483.1919, -719.0793)
  point P53 (556.085, -719.0793)
  point P54 (79.665, -1040.8293)
  point P55 (181.5581, -1069.8293)
  point P56 (108.665, -1069.8293)
  point P57 (254.4513, -1069.8293)
  point P58 (254.4513, -1069.8293)
  point P59 (108.665, -1069.8293)
  point P60 (108.665, -1069.8293)
  point P61 (254.4513, -1069.8293)
  point P62 (482.4419, -1069.8293)
  point P63 (555.335, -1069.8293)
  point P64 (555.335, -1069.8293)
  point P65 (409.5487, -1069.8293)
  point P66 (584.335, -1040.8293)
  point P67 (555.335, -1069.8293)
  point P68 (409.5487, -1069.8293)
  point P69 (409.5487, -1069.8293)
  dimension "d11" = 7
  dimension "d12" = 16.1835
  dimension "d13" = 16.1835
  dimension "d14" = 16.1835
  dimension "d15" = 16.1835
  dimension "d16" = 11.9217
  dimension "d17" = 11.9217
  dimension "d19" = 11.9217
  dimension "d22" = 5.3
  dimension "d23" = 5.3
  dimension "d24" = 5.3
  dimension "d25" = 5.3
  dimension "d26" = 5.3
  dimension "d27" = 22
  dimension "d28" = 22
  dimension "d29" = 22
  dimension "d33" = 5.3
  dimension "d34" = 5.3
  dimension "d35" = 5.3
  dimension "d36" = 5.3
  dimension "d37" = 5.3
  dimension "d38" = 5.3
  dimension "d39" = 5.3
  dimension "d43" = 291
  dimension "d63" = 74.7336
  dimension "d64" = 86
  dimension "d65" = 43
  dimension "d83" = 12.8931
  dimension "d84" = 12.8931
  dimension "d85" = 60
  dimension "d194" = 73
  dimension "d195" = 664
  dimension "d196" = 73
  dimension "d350" = 291
  dimension "d352" = 231
  dimension "d357" = 28.284
  dimension "d358" = 28.284
  dimension "d359" = 28.284
  dimension "d360" = 28.284
  dimension "d361" = 664
  dimension "d362" = 291
  dimension "d363" = 231
  dimension "d364" = 28.284
  dimension "d365" = 28.284
  dimension "d366" = 28.284
  dimension "d367" = 28.284
  dimension "d368" = 30
  dimension "d369" = 30
  dimension "d370" = 30
  dimension "d371" = 30
  dimension "d372" = 30
  dimension "d373" = 30
  dimension "d374" = 30
  dimension "d375" = 30
  dimension "d376" = 6.5
  dimension "d377" = 6.5
  dimension "d378" = 18
  dimension "d379" = 18
  dimension "d380" = 18
  dimension "d381" = 18
  dimension "d382" = 6.5
  dimension "d383" = 6.5
  dimension "d384" = 20
  dimension "d385" = 20
  dimension "d387" = 20
  dimension "d389" = 20
  dimension "d390" = 20
  dimension "d391" = 20
  dimension "d392" = 5
  dimension "d393" = 5
  dimension "d394" = 5
  dimension "d395" = 5
  dimension "d537" = 664
  dimension "d553" = 67
  dimension "d554" = 67
  dimension "d555" = 67
  dimension "d556" = 67
  dimension "d807" = 300
  dimension "d858" = 30
  dimension "d859" = 30
  dimension "d860" = 30
  dimension "d861" = 30
  dimension "d862" = 6.5
  dimension "d863" = 6.5
  dimension "d865" = 6.5
  dimension "d876" = 30
  dimension "d877" = 30
  dimension "d878" = 30
  dimension "d879" = 30
  dimension "d880" = 20
  dimension "d881" = 20
  dimension "d882" = 20
  dimension "d883" = 20
  dimension "d884" = 6.5
  dimension "d892" = 30
  dimension "d893" = 30
  dimension "d894" = 30
  dimension "d895" = 30
  dimension "d896" = 6.5
  dimension "d897" = 6.5
  dimension "d898" = 6.5
  dimension "d899" = 30
  dimension "d900" = 30
  dimension "d901" = 30
  dimension "d902" = 30
  dimension "d903" = 20
  dimension "d904" = 20
  dimension "d905" = 20
  dimension "d906" = 20
  dimension "d907" = 6.5
  dimension "d934" = 300
  dimension "d943" = 25
  dimension "d944" = 25
  dimension "d945" = 20
  dimension "d946" = 24.5
  dimension "d947" = 20
  dimension "d948" = 24.5
  dimension "d949" = 20
  dimension "d950" = 24.5
  dimension "d954" = 5
  dimension "d955" = 5
  dimension "d956" = 5
  dimension "d957" = 300
  dimension "d959" = 24.5
  dimension "d961" = 24.5
  dimension "d962" = 20
  dimension "d963" = 24.5
  dimension "d964" = 20
  dimension "d965" = 24.5
  dimension "d966" = 5
  dimension "d967" = 5
  dimension "d968" = 5
  dimension "d969" = 5
  dimension "d981" = 37.5
  dimension "d983" = 37.5
  dimension "d1011" = 8
  dimension "d1012" = 8
  dimension "d1013" = 8
  dimension "d1014" = 8
  dimension "d1015" = 8
  dimension "d1016" = 8
  dimension "d1017" = 8
  dimension "d1018" = 29
  dimension "d1019" = 45.5
  dimension "d1020" = 22
  dimension "d1049" = 182
  dimension "d1050" = 29
  dimension "d1051" = 45.5
  dimension "d1052" = 22
  dimension "d1055" = 2.5
  dimension "d1056" = 1.9
  dimension "d1057" = 273
  dimension "d1058" = 73
  dimension "d1059" = 8
  dimension "d1060" = 8
  dimension "d1061" = 8
  dimension "d1062" = 8
  dimension "d1063" = 8
  dimension "d1064" = 8
  dimension "d1065" = 8
  dimension "d1066" = 29
  dimension "d1069" = 182
  dimension "d1072" = 2.5
  dimension "d1073" = 1.9
  dimension "d1074" = 54.5
  dimension "d1075" = 26.5
  dimension "d1076" = 54.5
  dimension "d1077" = 17.5
  dimension "d1094" = 25
  dimension "d1095" = 25
  dimension "d1096" = 8
  dimension "d1097" = 8
  dimension "d1098" = 8
  dimension "d1099" = 8
  dimension "d1100" = 8
  dimension "d1101" = 8
  dimension "d1102" = 8
  dimension "d1103" = 29
  dimension "d1104" = 182
  dimension "d1105" = 2.5
  dimension "d1106" = 1.9
  dimension "d1107" = 54.5
  dimension "d1108" = 26.5
  dimension "d1109" = 54.5
  dimension "d1110" = 26.5
  dimension "d1111" = 8
  dimension "d1112" = 8
  dimension "d1113" = 8
  dimension "d1114" = 8
  dimension "d1115" = 8
  dimension "d1116" = 8
  dimension "d1117" = 8
  dimension "d1118" = 29
  dimension "d1119" = 45.5
  dimension "d1120" = 22
  dimension "d1121" = 182
  dimension "d1122" = 45.5
  dimension "d1123" = 22
  dimension "d1124" = 2.5
  dimension "d1125" = 1.9
  dimension "d1126" = 273
  dimension "d1127" = 73
  dimension "d1144" = 29
  dimension "d1145" = 29
  dimension "d1146" = 29
  dimension "d1147" = 29
  dimension "d1148" = 7
  dimension "d1171" = 291
  dimension "d1174" = 74.7336
  dimension "d1187" = 20
  dimension "d1188" = 20
  dimension "d1189" = 20
  dimension "d1190" = 20
  dimension "d1191" = 20
  dimension "d1192" = 20
  dimension "d1193" = 5
  dimension "d1194" = 5
  dimension "d1195" = 5
  dimension "d1196" = 5
  dimension "d1197" = 664
  dimension "d1210" = 29
  dimension "d1211" = 29
  dimension "d1212" = 29
  dimension "d1213" = 29
  dimension "d1237" = 291
  dimension "d1253" = 20
  dimension "d1254" = 20
  dimension "d1255" = 20
  dimension "d1256" = 20
  dimension "d1257" = 20
  dimension "d1258" = 20
  dimension "d1259" = 5
  dimension "d1260" = 5
  dimension "d1261" = 5
  dimension "d1262" = 5
  dimension "d1263" = 664
  dimension "d1322" = 29
  dimension "d1323" = 29
  dimension "d1324" = 12.5
  dimension "d1325" = 12.5
  dimension "d1326" = 58
  dimension "d1327" = 58
  dimension "d1328" = 58
  dimension "d1329" = 58
  dimension "d1330" = 58
  dimension "d1331" = 58
  dimension "d1332" = 12.8931
  dimension "d1333" = 12.8931
  dimension "d1334" = 60
  dimension "d1335" = 58
  dimension "d1336" = 58
  dimension "d1337" = 58
  dimension "d1338" = 58
  dimension "d1339" = 58
  dimension "d1340" = 58
  dimension "d1347" = 5.2
  constraint horizontal L0
  constraint horizontal L1
  constraint tangent L0 A0
  constraint tangent L1 A0
  constraint tangent L0 A1
  constraint tangent L1 A1
  constraint coincident L0.end A1.end
  constraint vertical L5
  constraint parallel L5 L6
  constraint parallel L6 L7
  constraint vertical L14
  constraint parallel L9 L14
  constraint parallel L9 L13
  constraint tangent A1 L15
  constraint horizontal L16
  constraint vertical L17
  constraint horizontal L19
  constraint vertical L20
  constraint coincident L17.end L18.start
  constraint coincident L20.end L21.end
  constraint coincident L4.end L5.start
  constraint coincident L7.end L8.end
  constraint coincident L22.start A7.centre
  constraint horizontal L23
  constraint parallel L23 L24
  constraint parallel L24 L25
  constraint horizontal L27
  constraint parallel L27 L28
  constraint parallel L28 L29
  constraint coincident L23.end L24.start
  constraint coincident L24.end L25.start
  constraint coincident L25.end A10.centre
  constraint coincident L26.start L27.start
  constraint coincident L27.end L28.start
  constraint coincident L28.end L29.start
  constraint coincident L29.end A14.centre
  constraint horizontal L30
  constraint vertical L31
  constraint horizontal L32
  constraint vertical L33
  constraint horizontal L34
  constraint vertical L35
  constraint vertical L36
  constraint perpendicular L35 L37
  constraint coincident A0.centre L37.end
  constraint horizontal L40
  constraint vertical L41
  constraint horizontal L42
  constraint vertical L43
  constraint horizontal L46
  constraint vertical L45
  constraint horizontal L47
  constraint vertical L44
  constraint horizontal L56
  constraint vertical L48
  constraint horizontal L50
  constraint vertical L49
  constraint horizontal L51
  constraint perpendicular L51 L53
  constraint parallel L51 L55
  constraint parallel L52 L53
  constraint coincident P1 L54
  constraint coincident P1 L57
  constraint coincident P1 P0
  constraint vertical L58
  constraint horizontal L68
  constraint vertical L66
  constraint horizontal L70
  constraint vertical L75
  constraint horizontal L74
  constraint perpendicular L72 L74
  constraint parallel L69 L74
  constraint parallel L65 L72
  constraint coincident P3 L71
  constraint coincident P3 L67
  constraint coincident P3 P2
  constraint vertical L77
  constraint coincident L57.start L51
  constraint coincident L57.start L53
  constraint tangent L51 A15
  constraint tangent L53 A15
  constraint coincident L54.start L51
  constraint coincident L54.start L52
  constraint tangent L51 A16
  constraint tangent L52 A16
  constraint coincident L57.end L52
  constraint coincident L57.end L55
  constraint tangent L52 A17
  constraint tangent L55 A17
  constraint coincident L54.end L53
  constraint coincident L54.end L55
  constraint tangent L53 A18
  constraint tangent L55 A18
  constraint coincident L67.start L74
  constraint coincident L67.start L72
  constraint tangent L74 A19
  constraint tangent L72 A19
  constraint coincident L71.start L74
  constraint coincident L71.start L65
  constraint tangent L74 A20
  constraint tangent L65 A20
  constraint coincident L67.end L65
  constraint coincident L67.end L69
  constraint tangent L65 A21
  constraint tangent L69 A21
  constraint coincident L71.end L72
  constraint coincident L71.end L69
  constraint tangent L72 A22
  constraint tangent L69 A22
  constraint coincident L64.end A23.centre
  constraint coincident L63.end A24.centre
  constraint coincident L59.end A25.centre
  constraint coincident L60.end A26.centre
  constraint coincident L61.end A27.centre
  constraint coincident L62.end A28.centre
  constraint coincident L76.end A29.centre
  constraint coincident L73.end A30.centre
  constraint horizontal L78
  constraint vertical L79
  constraint horizontal L80
  constraint vertical L81
  constraint horizontal L82
  constraint vertical L83
  constraint horizontal L84
  constraint vertical L85
  constraint horizontal L86
  constraint vertical L87
  constraint horizontal L88
  constraint vertical L89
  constraint horizontal L90
  constraint vertical L91
  constraint horizontal L92
  constraint vertical L93
  constraint coincident L91.end L92.start
  constraint coincident L79.end L80.start